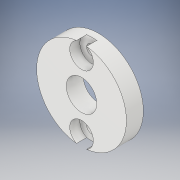
# Autodesk Inventor part: AA028
Saved by Autodesk Inventor 2017 SP1 (Build 210196100, 196)
## iProperties
Created: 2017-10-09
Part Number: AA028
Material: ABS Plastic
Document SubType Name: Modeling
Designer: Zach
Density: 1.06 g/cm^3
Appearance: CR White
Author: Zach
Autodesk Inventor part; units mm, degrees
ref_plane "YZ Plane" through (0, 0, 0) normal (1, 0, 0) x (0, 1, 0)
ref_plane "XZ Plane" through (0, 0, 0) normal (0, 1, 0) x (-1, 0, 0)
ref_plane "XY Plane" through (0, 0, 0) normal (0, 0, 1) x (1, 0, 0)
sketch "Sketch1" plane through (0, 0, 0) normal (0, 0, 1) x (1, 0, 0)
  circle A0 centre (0, 0) radius 13.25
  circle A1 centre (0, 0) radius 4.5
  dimension "d0" = 26.5
  dimension "d1" = 9
  constraints: 2 centre point, 2 coincident
  measures "d0" diameter of A0
  measures "d1" diameter of A1
extrude "Extrusion1" add sketch "Sketch1" along normal blind 5
sketch "Sketch2" plane through (0, 0, 5) normal (0, 0, 1) x (1, 0, 0)
  circle A0 centre (0, 10) radius 1.5
  circle A1 centre (0, -10) radius 1.5
  circle A2 centre (0, 0) radius 10 construction
  dimension "d4" = 3
  dimension "d5" = 3
  dimension "d6" = 20
  constraints: 3 centre point, 2 point on circle, 2 vertical alignment, 1 coincident
  measures "d4" diameter of A0
  measures "d5" diameter of A1
  measures "d6" diameter of A2
extrude "Extrusion2" cut sketch "Sketch2" against normal through all
sketch "Sketch3" plane through (0, 0, 5) normal (0, 0, 1) x (1, 0, 0)
  circle A0 centre (0, 10) radius 1.5 projected
  circle A1 centre (0, -10) radius 1.5 projected
  circle A2 centre (0, 10) radius 3.5
  circle A3 centre (0, -10) radius 3.5
  point P0 (0, 0)
  dimension "d9" = 7
  dimension "d10" = 7
  constraints: 2 centre point, 2 coincident
  measures "d9" diameter of A2
  measures "d10" diameter of A3
extrude "Extrusion3" cut sketch "Sketch3" against normal blind 3
body "Solid1"
